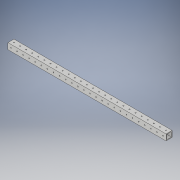
# Autodesk Inventor part: numbah 9
Saved by Autodesk Inventor 2018 (Build 220112000, 112)
## iProperties
Created: 2018-02-03
Part Number: numbah 9
Material: Generic
Document SubType Name: Modeling
Designer: matuch.michael
Density: 1 g/cm^3
Appearance: Default
Author: matuch.michael
Autodesk Inventor part; units mm, degrees
ref_plane "YZ Plane" through (0, 0, 0) normal (1, 0, 0) x (0, 1, 0)
ref_plane "XZ Plane" through (0, 0, 0) normal (0, 1, 0) x (-1, 0, 0)
ref_plane "XY Plane" through (0, 0, 0) normal (0, 0, 1) x (1, 0, 0)
sketch "Sketch1" plane through (0, 0, 0) normal (0, 0, 1) x (1, 0, 0)
  line L0 (-5.91, 5.4476) -> (654.49, 5.4476)
  line L1 (654.49, 5.4476) -> (654.49, -19.9524)
  line L2 (654.49, -19.9524) -> (-5.91, -19.9524)
  line L3 (-5.91, -19.9524) -> (-5.91, 5.4476)
  point P0 (0, 0)
  dimension "d0" = 660.4
  dimension "d1" = 25.4
  constraints: 8 end point, 2 parallel, 1 horizontal, 1 perpendicular
  measures "d0" distance of L1.end L2.end
  measures "d1" distance of L0.end L1.end
extrude "Extrusion1" add sketch "Sketch1" along normal blind 25.4
sketch "Sketch2" plane through (0, 0, 25.4) normal (0, 0, 1) x (1, 0, 0)
  circle A0 centre (6.79, -7.2524) radius 1.9685
  line L0 (-5.91, 5.4476) -> (-5.91, -19.9524) projected
  line L1 (-5.91, -19.9524) -> (654.49, -19.9524) projected
  circle A1 centre (32.19, -7.2524) radius 1.9685
  circle A2 centre (57.59, -7.2524) radius 1.9685
  circle A3 centre (82.99, -7.2524) radius 1.9685
  circle A4 centre (108.39, -7.2524) radius 1.9685
  circle A5 centre (133.79, -7.2524) radius 1.9685
  circle A6 centre (159.19, -7.2524) radius 1.9685
  circle A7 centre (184.59, -7.2524) radius 1.9685
  circle A8 centre (209.99, -7.2524) radius 1.9685
  circle A9 centre (235.39, -7.2524) radius 1.9685
  circle A10 centre (260.79, -7.2524) radius 1.9685
  circle A11 centre (286.19, -7.2524) radius 1.9685
  circle A12 centre (311.59, -7.2524) radius 1.9685
  circle A13 centre (336.99, -7.2524) radius 1.9685
  circle A14 centre (362.39, -7.2524) radius 1.9685
  circle A15 centre (387.79, -7.2524) radius 1.9685
  circle A16 centre (413.19, -7.2524) radius 1.9685
  circle A17 centre (438.59, -7.2524) radius 1.9685
  circle A18 centre (463.99, -7.2524) radius 1.9685
  circle A19 centre (489.39, -7.2524) radius 1.9685
  circle A20 centre (514.79, -7.2524) radius 1.9685
  circle A21 centre (540.19, -7.2524) radius 1.9685
  circle A22 centre (565.59, -7.2524) radius 1.9685
  circle A23 centre (590.99, -7.2524) radius 1.9685
  circle A24 centre (616.39, -7.2524) radius 1.9685
  circle A25 centre (641.79, -7.2524) radius 1.9685
  point P0 (0, 0)
  dimension "d4" = 3.937
  dimension "d5" = 12.7
  dimension "d6" = 12.7
  dimension "d9" = 25.4
  dimension "d16" = 25.4
  constraints: 26 centre point, 2 horizontal, 50 other
  measures "d4" diameter of A0
  measures "d5" distance from line of L0 A0.centre
  measures "d6" distance from line of L1 A0.centre
  measures "d9" distance of A0.centre A1.centre
  measures "d16" distance of A24.centre A25.centre
extrude "Extrusion2" cut sketch "Sketch2" against normal blind 25.4
sketch "Sketch3" plane through (-5.91, -19.9524, 0) normal (-1, 0, 0) x (0, 0, 1)
  line L0 (3.175, 22.225) -> (22.225, 22.225)
  line L1 (22.225, 22.225) -> (22.225, 3.175)
  line L2 (22.225, 3.175) -> (3.175, 3.175)
  line L3 (3.175, 3.175) -> (3.175, 22.225)
  line L4 (0, 25.4) -> (25.4, 25.4) projected
  line L5 (0, 0) -> (0, 25.4) projected
  line L6 (0, 0) -> (25.4, 0) projected
  line L7 (25.4, 25.4) -> (25.4, 0) projected
  point P0 (0, 19.9524)
  dimension "d23" = 3.175
  dimension "d24" = 3.175
  dimension "d25" = 3.175
  dimension "d26" = 3.175
  constraints: 8 end point, 2 parallel, 1 horizontal, 1 perpendicular
  measures "d23" distance between parallel lines of L4 L0
  measures "d24" distance between parallel lines of L5 L3
  measures "d25" distance between parallel lines of L6 L2
  measures "d26" distance between parallel lines of L7 L1
sketch "Sketch4" plane through (-5.91, 5.4476, 0) normal (0, 1, 0) x (1, 0, 0)
  circle A0 centre (12.7, -12.7) radius 1.9685
  line L0 (0, 0) -> (0, -25.4) projected
  line L1 (660.4, -25.4) -> (0, -25.4) projected
  circle A1 centre (38.1, -12.7) radius 1.9685
  circle A2 centre (63.5, -12.7) radius 1.9685
  circle A3 centre (88.9, -12.7) radius 1.9685
  circle A4 centre (114.3, -12.7) radius 1.9685
  circle A5 centre (139.7, -12.7) radius 1.9685
  circle A6 centre (165.1, -12.7) radius 1.9685
  circle A7 centre (190.5, -12.7) radius 1.9685
  circle A8 centre (215.9, -12.7) radius 1.9685
  circle A9 centre (241.3, -12.7) radius 1.9685
  circle A10 centre (266.7, -12.7) radius 1.9685
  circle A11 centre (292.1, -12.7) radius 1.9685
  circle A12 centre (317.5, -12.7) radius 1.9685
  circle A13 centre (342.9, -12.7) radius 1.9685
  circle A14 centre (368.3, -12.7) radius 1.9685
  circle A15 centre (393.7, -12.7) radius 1.9685
  circle A16 centre (419.1, -12.7) radius 1.9685
  circle A17 centre (444.5, -12.7) radius 1.9685
  circle A18 centre (469.9, -12.7) radius 1.9685
  circle A19 centre (495.3, -12.7) radius 1.9685
  circle A20 centre (520.7, -12.7) radius 1.9685
  circle A21 centre (546.1, -12.7) radius 1.9685
  circle A22 centre (571.5, -12.7) radius 1.9685
  circle A23 centre (596.9, -12.7) radius 1.9685
  circle A24 centre (622.3, -12.7) radius 1.9685
  circle A25 centre (647.7, -12.7) radius 1.9685
  point P0 (5.91, 0)
  dimension "d27" = 3.937
  dimension "d28" = 12.7
  dimension "d29" = 12.7
  dimension "d32" = 25.4
  constraints: 26 centre point, 1 horizontal, 50 other
  measures "d27" diameter of A0
  measures "d28" distance from line of L0 A0.centre
  measures "d29" distance from line of L1 A0.centre
  measures "d32" distance of A0.centre A1.centre
extrude "Extrusion3" cut sketch "Sketch4" against normal blind 25.4
extrude "Extrusion4" cut sketch "Sketch3" against normal blind 660.4 contours L0 L1 L2 L3
body "Solid1"
